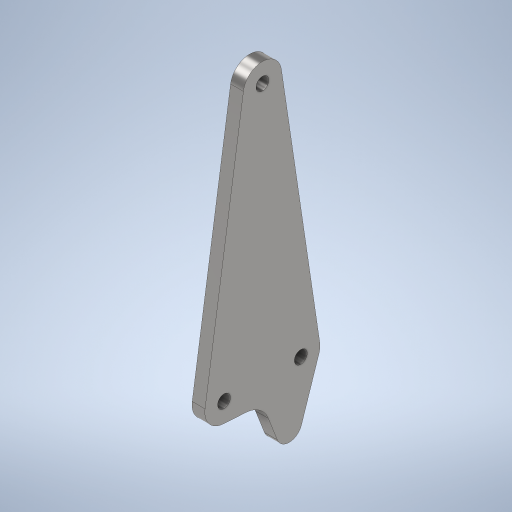
# Autodesk Inventor part: Anti-inverter
Saved by Autodesk Inventor 2023 (Build 270158000, 158)
## iProperties
Created: 2023-01-16
Part Number: Anti-inverter
Material: Steel, Carbon
Document SubType Name: Modeling
Designer: justi
Density: 7.85 g/cm^3
Appearance: Semi-Polished
Mass: 297.596 g
Surface Area: 148.387 cm^2
Volume: 37.9104 cm^3
Author: justi
Autodesk Inventor part; units mm, degrees
ref_plane "YZ Plane" through (0, 0, 0) normal (1, 0, 0) x (0, 1, 0)
ref_plane "XZ Plane" through (0, 0, 0) normal (0, 1, 0) x (-1, 0, 0)
ref_plane "XY Plane" through (0, 0, 0) normal (0, 0, 1) x (1, 0, 0)
sketch "Sketch2" plane through (0, 0, 0) normal (1, 0, 0) x (0, 1, 0)
  circle A0 centre (0, 0) radius 3.175
  circle A1 centre (0, -38.1) radius 3.175
  circle A2 centre (0, 0) radius 9.525
  circle A3 centre (0, -38.1) radius 9.525
  line L0 (-9.525, 0) -> (9.525, 0)
  line L1 (9.525, 0) -> (9.525, -38.1)
  line L2 (9.525, -38.1) -> (-9.525, -38.1)
  line L3 (-9.525, -38.1) -> (-9.525, 0)
  line L4 (0, -19.05) -> (-25.4, -19.05)
  line L5 (-25.4, -19.05) -> (-7.7378, 5.5545)
  line L6 (-25.4, -19.05) -> (-7.7378, -43.6545)
  line L7 (0, -19.05) -> (127, -19.05)
  circle A4 centre (127, -19.05) radius 3.175
  circle A5 centre (127, -19.05) radius 9.525
  line L8 (127, -19.05) -> (0, 0)
  line L9 (0, 0) -> (1.4129, 9.4196)
  line L10 (1.4129, 9.4196) -> (128.4129, -9.6304)
  line L11 (128.4129, -9.6304) -> (127, -19.05)
  line L12 (0, -38.1) -> (127, -19.05)
  line L13 (127, -19.05) -> (128.4129, -28.4696)
  line L14 (128.4129, -28.4696) -> (1.4129, -47.5196)
  line L15 (1.4129, -47.5196) -> (0, -38.1)
  line L16 (0, 0) -> (0, -38.1)
  point P0 (1.4129, 9.4196)
  point P1 (1.4129, -47.5196)
  point P2 (128.4129, -28.4696)
  point P3 (128.4129, -9.6304)
  dimension "d11" = 6.35
  dimension "d12" = 6.35
  dimension "d13" = 38.1
  dimension "d14" = 19.05
  dimension "d15" = 19.05
  dimension "d16" = 25.4
  dimension "d17" = 127
  dimension "d18" = 180
  dimension "d19" = 6.35
  dimension "d20" = 19.05
  dimension "d21" = 9.525
  dimension "d22" = 9.525
  constraints: 34 end point, 6 centre point, 6 parallel, 5 coincident, 4 point on circle, 3 perpendicular, 2 horizontal, 2 tangent
  measures "d11" diameter of A0
  measures "d12" diameter of A1
  measures "d13" distance of point (0, 0) A1.centre
  measures "d14" diameter of A2
  measures "d15" diameter of A3
  measures "d16" distance of L4.start L4.end
  measures "d17" distance of L4.start L7.end
  measures "d18" angle of L4 L7
  measures "d19" diameter of A4
  measures "d20" diameter of A5
  measures "d21" distance of L8.start L13.end
  measures "d22" distance of L10.end L8.start
extrude "Extrusion2" add sketch "Sketch2" along normal blind 6.35 contours L0 A2 L8 A0 | A0 L9 A2 L0 | A0 L0 A2 L9 | L8 A2 L16 A0 | L1 L8 A2 | A2 L10 A5 L8 L1 | A0 L16 A2 L0 | L8 L1 L7 L16 A2 | L8 A5 L7 L1 | L3 L4 L5 A2 | A2 L16 L4 L3 | L11 A4 L8 A5 | A5 L13 A4 L11 | L7 A5 L12 L1 | L1 L12 A3 L16 L7 | L8 A4 L7 A5 | L4 L16 A3 L3 | L3 A3 L6 L4 | L12 A5 L14 A3 L1 | L1 A3 L12 | L7 A4 L12 A5 | L2 A1 L15 A3 | A3 L16 A1 L2 | A5 L12 A4 L13 | A3 L12 A1 L16 | L2 A1 L12 A3 | A3 L15 A1 L2
fillet "Fillet1" radius 41.275 1 edges at (3.175, -25.4, -19.05)
sketch "Sketch4" plane through (6.35, 0, 0) normal (1, 0, 0) x (0, 0, -1)
  circle A0 centre (0, 0) radius 3.175 projected
  circle A1 centre (0, 0) radius 9.525
  circle A2 centre (38.1, 0) radius 3.175 projected
  circle A3 centre (38.1, 0) radius 9.525
  line L0 (19.05, 0) -> (19.05, -10.795)
  line L1 (19.05, -10.795) -> (-0.6234, -9.5046)
  line L2 (19.05, -10.795) -> (39.6075, -9.405)
  line L3 (-5.5545, -7.7378) -> (-5.0196, -8.1218) projected
  line L4 (-5.5545, -7.7378) -> (23.2464, -38.8808)
  line L5 (23.2464, -38.8808) -> (43.6545, -7.7378)
  line L6 (0, 0) -> (38.1, 0)
  dimension "d26" = 19.05
  dimension "d27" = 19.05
  dimension "d28" = 10.795
  dimension "d29" = 19.05
  dimension "d38" = 0
  constraints: 12 end point, 3 point on circle, 2 centre point, 2 coincident, 1 horizontal, 1 tangent, 1 vertical
  measures "d26" diameter of A1
  measures "d27" diameter of A3
  measures "d28" distance of L0.start L0.end
  measures "d29" distance from line of L6.start L0
  measures "d38" distance from line of L6 L0.start
extrude "Extrusion3" cut sketch "Sketch4" against normal blind 6.35 contours A1 L1 L2 A3 L5 L4 | L2 A3 picked at (38.8374, -9.4689)
sketch "Sketch5" plane through (6.35, 0, 0) normal (1, 0, 0) x (0, 0, -1)
  line L0 (39.6075, -9.405) -> (19.05, -10.795) projected
  line L1 (19.05, -10.795) -> (32.8572, -46.3052)
  line L2 (32.8572, -46.3052) -> (47.1457, -2.9835)
  arc A0 (39.6075, -9.405) -> (47.5196, 1.4129) centre (38.1, 0) ccw projected
  line L3 (-0.6234, -9.5046) -> (19.05, -10.795) projected
  circle A1 centre (38.1, 0) radius 9.525
  line L4 (19.05, -10.795) -> (-0.6234, -9.5046) projected
  line L5 (19.3477, -12.6523) -> (39.6075, -9.405)
  point P0 (0, 0)
  dimension "d32" = 38.1
  dimension "d33" = 115
  constraints: 6 end point, 3 tangent, 1 centre point, 1 coincident, 1 concentric, 1 point on circle
  measures "d32" distance of L0.end L1.end
  measures "d33" angle of L1 L3
extrude "Extrusion4" add sketch "Sketch5" against normal blind 6.35 contours A1 L0 | L5 L1 L0 A1 | A0 L2 L1 L5
fillet "Fillet2" radius 6.35 1 edges at (3.175, -46.3052, -32.8572)
fillet "Fillet3" radius 12.7 1 edges at (3.175, -10.795, -19.05)
body "Solid2"
